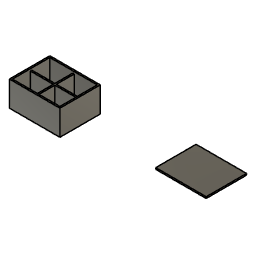
10403김동현_보관함 v1 (Autodesk Fusion 360 design; units mm, degrees)
Autodesk Fusion 360 part; units mm, degrees
sketch "스케치1" plane through (0, 0, 0) normal (0, 0, 1) x (1, 0, 0)
  line L0 (-50, 40) -> (50, 40)
  line L1 (50, 40) -> (50, -40)
  line L2 (50, -40) -> (-50, -40)
  line L3 (-50, -40) -> (-50, 40)
  line L4 (-50, 40) -> (50, -40) construction
  dimension "d3" = 100
  dimension "d4" = 80
  constraint horizontal L0
  constraint vertical L1
  constraint horizontal L2
  constraint vertical L3
  constraint midpoint origin L4
  measures "d3" distance of L0.start L0.end
  measures "d4" distance of L0.start L2.end
extrude "돌출1" add sketch "스케치1" along normal blind 50 makes body 1
shell "쉘1" thickness 3 removed faces 1 at (-16.6667, 13.3333, 50) on bodies 1
sketch "스케치2" plane through (0, 0, 3) normal (0, 0, 1) x (-1, 0, 0)
  line L0 (47, -1.5) -> (-47, -1.5)
  line L1 (-47, -1.5) -> (-47, 1.5)
  line L2 (-47, 1.5) -> (47, 1.5)
  line L3 (47, 1.5) -> (47, -1.5)
  line L4 (47, -1.5) -> (-47, 1.5) construction
  line L5 (1.5, -37) -> (-1.5, -37)
  line L6 (-1.5, -37) -> (-1.5, 37)
  line L7 (-1.5, 37) -> (1.5, 37)
  line L8 (1.5, 37) -> (1.5, -37)
  line L9 (47, -37) -> (-47, -37)
  line L10 (-47, 37) -> (47, 37)
  line L11 (1.5, -37) -> (-1.5, 37) construction
  dimension "d9" = 3
  dimension "d10" = 94
  dimension "d11" = 3
  dimension "d13" = 3
  dimension "d14" = 74
  constraint horizontal L0
  constraint vertical L1
  constraint horizontal L2
  constraint vertical L3
  constraint midpoint origin L4
  constraint horizontal L5
  constraint vertical L6
  constraint horizontal L7
  constraint vertical L8
  constraint coincident L6.end L10
  constraint coincident L5.start L9
  constraint midpoint origin L11
  measures "d9" distance of L0.end L1.end
  measures "d10" distance of L0.start L0.end
  measures "d11" distance of L6.end L7.end
  measures "d13" distance of L5.start L5.end
  measures "d14" distance of L5.start L7.end
extrude "돌출2" add sketch "스케치2" along normal blind 43 bodies 1
sketch "스케치3" plane through (0, 0, 0) normal (0, 0, 1) x (1, 0, 0)
  line L0 (200, 80) -> (300, 80)
  line L1 (300, 80) -> (300, 0)
  line L2 (300, 0) -> (200, 0)
  line L3 (200, 0) -> (200, 80)
  dimension "d17" = 100
  dimension "d18" = 80
  constraint horizontal L0
  constraint vertical L1
  constraint horizontal L2
  constraint vertical L3
  measures "d17" distance of L1.end L2.end
  measures "d18" distance of L0.start L2.end
extrude "돌출3" add sketch "스케치3" along normal blind 3 separate body makes body 2
sketch "스케치4" plane through (0, 0, 0) normal (0, 0, 1) x (1, 0, 0)
  line L0 (203, 77) -> (297, 77)
  line L1 (297, 77) -> (297, 3)
  line L2 (297, 3) -> (203, 3)
  line L3 (203, 3) -> (203, 77)
  line L4 (300, 0) -> (300, 80)
  line L5 (300, 80) -> (200, 80)
  dimension "d21" = 74
  dimension "d22" = 94
  dimension "d23" = 74
  dimension "d24" = 3
  dimension "d25" = 3
  constraint horizontal L0
  constraint vertical L1
  constraint horizontal L2
  constraint vertical L3
  measures "d21" distance of L0.end L1.end
  measures "d22" distance of L0.start L0.end
  measures "d23" distance of L0.start L2.end
  measures "d24" distance of L1 L4
  measures "d25" distance of L0 L5
extrude "돌출4" add sketch "스케치4" against normal blind 3 bodies 2
